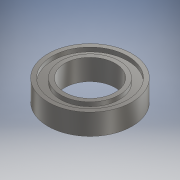
# Autodesk Inventor part: bearing_6x10x2,5
Saved by Autodesk Inventor 2017 (Build 210142000, 142)
## iProperties
Created: 2017-02-09
Part Number: bearing_6x10x2,5
Material: Stainless Steel
Document SubType Name: Modeling
Designer: JT
Density: 8 g/cm^3
Appearance: Semi-Polished
Author: JT
Autodesk Inventor part; units mm, degrees
ref_plane "YZ Plane" through (0, 0, 0) normal (1, 0, 0) x (0, 1, 0)
ref_plane "XZ Plane" through (0, 0, 0) normal (0, 1, 0) x (-1, 0, 0)
sketch "Sketch1" plane through (0, 0, 0) normal (0, 0, 1) x (1, 0, 0)
  circle A0 centre (0, 0) radius 5
  dimension "d0" = 10
  constraints: 1 centre point, 1 coincident
  measures "d0" diameter of A0
extrude "Extrusion1" add sketch "Sketch1" along normal blind 2.5
hole "Hole1" at (0, 0, 2.5) direction (0, 0, -1) diameter 6 end through all
sketch "Sketch2" plane through (0, 0, 2.5) normal (0, 0, 1) x (1, 0, 0)
  circle A0 centre (0, 0) radius 4.5
  circle A1 centre (0, 0) radius 3.5
  dimension "d12" = 9
  dimension "d13" = 7
  constraints: 2 centre point, 2 coincident
  measures "d12" diameter of A0
  measures "d13" diameter of A1
extrude "Extrusion2" cut sketch "Sketch2" against normal blind 0.5
ref_plane "Work Plane1" through (0, 0, 1.25) normal (0, 0, 1) x (1, 0, 0)
mirror "Mirror1" about plane through (0, 0, 1.25) normal (0, 0, 1) of "Extrusion2"
body "Solid1"
